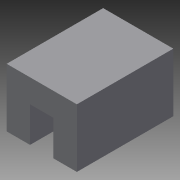
# Autodesk Inventor part: Roller ver2
Saved by Autodesk Inventor 2015 (Build 190159000, 159)
## iProperties
Created: 2016-05-27
Part Number: Roller ver2
Material: Generic
Document SubType Name: Modeling
Designer: Toby
Density: 1 g/cm^3
Appearance: Default
Author: Toby
Autodesk Inventor part; units mm, degrees
ref_plane "YZ Plane" through (0, 0, 0) normal (1, 0, 0) x (0, 1, 0)
ref_plane "XZ Plane" through (0, 0, 0) normal (0, 1, 0) x (-1, 0, 0)
ref_plane "XY Plane" through (0, 0, 0) normal (0, 0, 1) x (1, 0, 0)
sketch "Sketch1" plane through (0, 0, 0) normal (0, 0, 1) x (1, 0, 0)
  line L0 (-9.1129, 4.4946) -> (-3.1129, 4.4946)
  line L1 (-3.1129, 4.4946) -> (-3.1129, -3.7524)
  line L2 (-3.1129, -3.7524) -> (-9.1129, -3.7524)
  line L3 (-9.1129, -3.7524) -> (-9.1129, 4.4946)
  line L4 (-9.1129, 4.4946) -> (-7.1129, 4.4946)
  line L5 (-7.1129, 4.4946) -> (-7.1129, -3.7524)
  line L6 (-7.1129, -3.7524) -> (-9.1129, -3.7524)
  line L7 (-9.1129, -3.7524) -> (-9.1129, 4.4946)
  line L8 (-3.1129, 4.4946) -> (-5.1129, 4.4946)
  line L9 (-5.1129, 4.4946) -> (-5.1129, -3.7524)
  line L10 (-5.1129, -3.7524) -> (-3.1129, -3.7524)
  line L11 (-3.1129, -3.7524) -> (-3.1129, 4.4946)
  point P0 (0, 0)
  dimension "d0" = 6
  dimension "d1" = 2
  dimension "d2" = 2
  constraints: 24 end point, 6 parallel, 3 horizontal, 3 perpendicular, 2 point on line
  measures "d0" distance of L0.start L0.end
  measures "d1" distance between parallel lines of L3 L5
  measures "d2" distance between parallel lines of L1 L9
extrude "Extrusion1" add sketch "Sketch1" along normal blind 5 contours L0 L5 L2 L3 | L0 L1 L2 L9
sketch "Sketch2" plane through (0, 0, 5) normal (0, 0, 1) x (1, 0, 0)
  line L0 (-9.1129, 4.4946) -> (-3.1129, 4.4946)
  line L1 (-3.1129, 4.4946) -> (-3.1129, -3.7524)
  line L2 (-3.1129, -3.7524) -> (-9.1129, -3.7524)
  line L3 (-9.1129, -3.7524) -> (-9.1129, 4.4946)
  point P0 (0, 0)
  constraints: 8 end point, 2 parallel, 1 horizontal, 1 perpendicular
extrude "Extrusion2" add sketch "Sketch2" against normal blind 2
body "Solid1"
